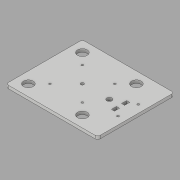
# Autodesk Inventor part: E_base1
Saved by Autodesk Inventor 2019 (Build 230136000, 136)
## iProperties
Created: 2021-11-01
Part Number: E_base1
Material: Generic
Document SubType Name: Modeling
Designer: Mohamed
Density: 1 g/cm^3
Appearance: Default
Author: Mohamed
Autodesk Inventor part; units mm, degrees
ref_plane "YZ Plane" through (0, 0, 0) normal (1, 0, 0) x (0, 1, 0)
ref_plane "XZ Plane" through (0, 0, 0) normal (0, 1, 0) x (-1, 0, 0)
ref_plane "XY Plane" through (0, 0, 0) normal (0, 0, 1) x (1, 0, 0)
sketch "Sketch1" plane through (0, 0, 0) normal (0, 1, 0) x (-1, 0, 0)
  line L0 (5, 0) -> (145, 0)
  line L1 (150, -5) -> (150, -145)
  line L2 (145, -150) -> (5, -150)
  line L3 (0, -145) -> (0, -5)
  arc A0 (150, -5) -> (145, 0) centre (145, -5) ccw
  arc A1 (150, -5) -> (145, 0) centre (145, -5) ccw
  arc A2 (145, -150) -> (150, -145) centre (145, -145) ccw
  arc A3 (5, 0) -> (0, -5) centre (5, -5) ccw
  arc A4 (0, -145) -> (5, -150) centre (5, -145) ccw
  circle A5 centre (128.033, -21.967) radius 9.5
  circle A6 centre (128.033, -128.033) radius 9.5
  circle A7 centre (21.967, -128.033) radius 9.5
  circle A8 centre (21.967, -21.967) radius 9.5
  circle A9 centre (21.967, -75) radius 5
  point P0 (150, -150)
  point P1 (150, 0)
  point P2 (0, -150)
  dimension "d12" = 150
  dimension "d13" = 150
  dimension "d22" = 5
  dimension "d23" = 5
  dimension "d28" = 19
  dimension "d29" = 19
  dimension "d30" = 19
  dimension "d31" = 19
  dimension "d32" = 10
  constraints: 10 centre point, 10 point on circle, 10 tangent, 8 end point, 8 point on line, 3 equal radius, 2 parallel, 1 horizontal, 1 perpendicular
  measures "d12" distance of point (150, -150) point (0, -150)
  measures "d13" distance of point (150, 0) point (150, -150)
  measures "d22" radius of A0
  measures "d23" radius of A2
  measures "d28" diameter of A5
  measures "d29" diameter of A6
  measures "d30" diameter of A7
  measures "d31" diameter of A8
  measures "d32" diameter of A9
extrude "Extrusion1" add sketch "Sketch1" along normal blind 6
sketch "Sketch2" plane through (0, 6, 0) normal (0, 1, 0) x (1, 0, 0)
  circle A0 centre (-128.033, 21.967) radius 9.5 projected
  circle A1 centre (-21.967, 128.033) radius 9.5 projected
  circle A2 centre (-128.033, 128.033) radius 9.5 projected
  circle A3 centre (-75, 75) radius 3
  circle A4 centre (-21.967, 21.967) radius 9.5 projected
  circle A5 centre (-106.8198, 43.1802) radius 2
  circle A6 centre (-43.1802, 43.1802) radius 2
  circle A7 centre (-43.1802, 106.8198) radius 2
  circle A8 centre (-106.8198, 106.8198) radius 2
  point P0 (0, 0)
  dimension "d35" = 6
  dimension "d40" = 4
  dimension "d41" = 4
  dimension "d42" = 4
  dimension "d43" = 4
  dimension "d47" = 30
  constraints: 5 centre point
  measures "d35" diameter of A3
  measures "d40" diameter of A5
  measures "d41" diameter of A6
  measures "d42" diameter of A7
  measures "d43" diameter of A8
  measures "d47" distance of A8.centre A2.centre
extrude "Extrusion2" cut sketch "Sketch2" against normal blind 6 contours A3 | A5 | A6 | A7 | A8
sketch "Sketch3" plane through (0, 6, 0) normal (0, 1, 0) x (1, 0, 0)
  arc A0 (-5, 0) -> (0, 5) centre (-5, 5) ccw projected
  line L0 (-5, 0) -> (25, 0)
  line L1 (30, 5) -> (30, 145)
  line L2 (25, 150) -> (-5, 150)
  line L3 (-5, 150) -> (-5, 0)
  arc A1 (25, 0) -> (30, 5) centre (25, 5) ccw
  arc A2 (30, 145) -> (25, 150) centre (25, 145) ccw
  point P0 (0, 0)
  point P1 (30, 150)
  point P2 (30, 0)
  dimension "d48" = 35
  dimension "d49" = 150
  dimension "d50" = 5
  constraints: 8 end point, 4 point on circle, 4 point on line, 4 tangent, 2 centre point, 2 parallel, 1 equal radius, 1 horizontal, 1 perpendicular
  measures "d48" distance of L2.end point (30, 150)
  measures "d49" distance of point (30, 150) point (30, 0)
  measures "d50" radius of A1
extrude "Extrusion3" add sketch "Sketch3" against normal blind 6
sketch "Sketch4" plane through (0, 6, 0) normal (0, 1, 0) x (1, 0, 0)
  line L0 (30, 5) -> (30, 145) projected
  circle A0 centre (15, 55) radius 2.1
  circle A1 centre (15, 95) radius 2.1
  line L1 (-3, 80) -> (3, 80)
  line L2 (3, 80) -> (3, 90)
  line L3 (3, 90) -> (-3, 90)
  line L4 (-3, 90) -> (-3, 80)
  line L5 (-3, 70) -> (3, 70)
  line L6 (3, 70) -> (3, 60)
  line L7 (3, 60) -> (-3, 60)
  line L8 (-3, 60) -> (-3, 70)
  line L9 (15, 75) -> (15, 55)
  line L10 (15, 75) -> (15, 95)
  point P0 (0, 0)
  dimension "d55" = 4.2
  dimension "d56" = 4.2
  dimension "d58" = 10
  dimension "d60" = 6
  dimension "d61" = 10
  dimension "d62" = 6
  dimension "d63" = 10
  dimension "d67" = 20
  dimension "d68" = 20
  constraints: 20 end point, 4 parallel, 2 centre point, 2 horizontal, 2 perpendicular, 1 vertical
  measures "d55" diameter of A0
  measures "d56" diameter of A1
  measures "d58" distance of L5.start L1.start
  measures "d60" distance of L3.end L2.end
  measures "d61" distance of L2.end L1.end
  measures "d62" distance of L6.end L7.end
  measures "d63" distance of L5.end L6.end
  measures "d67" distance of L9.start L9.end
  measures "d68" distance of L9.start L10.end
extrude "Extrusion4" cut sketch "Sketch4" against normal blind 6
body "Solid1"
